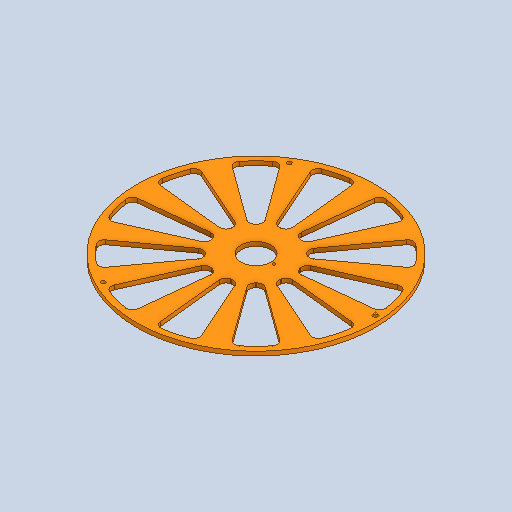
# Autodesk Inventor part: torsosc-electrode-pcb-fr4
Saved by Autodesk Inventor 2026 (Build 300175050, 175E)
## iProperties
Created: 2021-01-06
Part Number: torsosc-electrode-pcb-fr4
Material: Epoxy Resin
Document SubType Name: Modeling
Designer: schanen
Density: 1.14 g/cm^3
Appearance: Orange
Author: schanen
Autodesk Inventor part; units mm, degrees
ref_plane "YZ Plane" through (0, 0, 0) normal (1, 0, 0) x (0, 1, 0)
ref_plane "XZ Plane" through (0, 0, 0) normal (0, 1, 0) x (-1, 0, 0)
ref_plane "XY Plane" through (0, 0, 0) normal (0, 0, 1) x (1, 0, 0)
sketch "Sketch1" plane through (0, 0, 0) normal (0, 1, 0) x (-1, 0, 0)
  circle A0 centre (0, 0) radius 20
  circle A1 centre (0, 0) radius 2.5
  dimension "d0" = 40
  dimension "d1" = 5
  constraints: 2 centre point, 2 coincident
  measures "d0" diameter of A0
  measures "d1" diameter of A1
extrude "Extrusion1" add sketch "Sketch1" along normal blind 0.7
sketch "Sketch5" plane through (0, 0.7, 0) normal (0, 1, 0) x (1, 0, 0)
  circle A0 centre (0, 0) radius 19 construction
  point P0 (18.974, 0.9944)
  point P1 (19, 0)
  dimension "d35" = 38
  dimension "d36" = 3
  constraints: 2 point on circle, 1 centre point, 1 coincident, 1 horizontal alignment
  measures "d35" diameter of A0
hole "Hole3" at (18.974, 0.7, -0.9944) direction (0, -1, 0) diameter 0.7 end through all
pattern_circular "Circular Pattern1" count 3 over 360 about axis through (0, -10, 0) along (0, 1, 0) of "Hole3"
sketch "Sketch6" plane through (0, 0.7, 0) normal (0, 1, 0) x (1, 0, 0)
  circle A0 centre (0, 0) radius 6
  line L0 (0, 0) -> (-1.986, 18.8959)
  line L1 (0, 0) -> (-7.728, 17.3574)
  line L2 (0, 28) -> (0, -28) projected
  circle A1 centre (0, 0) radius 19
  point P0 (-2.4404, 5.4813)
  point P1 (-0.6272, 5.9671)
  dimension "d47" = 12
  dimension "d51" = 38
  dimension "d53" = 6
  dimension "d54" = 18
  constraints: 4 end point, 2 centre point, 2 coincident, 2 point on circle
  measures "d47" diameter of A0
  measures "d51" diameter of A1
  measures "d53" angle of L2 L0
  measures "d54" angle of L0 L1
extrude "Extrusion3" cut sketch "Sketch6" against normal through all contours A0 L1 A1 L0
fillet "Fillet1" radius 1 4 edges at (-7.728, 0.35, -17.3574) (-1.986, 0.35, -18.8959) (-2.4404, 0.35, -5.4813) (-0.6272, 0.35, -5.9671)
pattern_circular "Circular Pattern2" count 12 over 360 about axis through (0, 0, 0) along (0, 1, 0) of "Extrusion3", "Fillet1"
sketch "Sketch7" plane through (0, 0.7, 0) normal (0, 1, 0) x (1, 0, 0)
  point P0 (0, 0)
  point P1 (3, 0)
  dimension "d61" = 3
  measures "d61" distance of point (0, 0) point (3, 0)
hole "Hole4" at (3, 0.7, 0) direction (0, -1, 0) diameter 0.5 end through all
body "Solid1"
